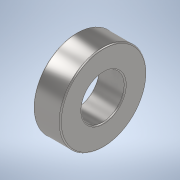
# Autodesk Inventor part: 608zz-bearing
Saved by Autodesk Inventor 2020 (Build 240168000, 168)
## iProperties
Created: 2021-03-01
Part Number: 608zz-bearing
Material: Steel, Carbon
Document SubType Name: Modeling
Designer: AOB
Mass: 5.9086 g
Surface Area: 6.6564 cm^2
Volume: 0.752688 cm^3
Density: 7.85 g/cm^3
Appearance: Semi-Polished
Author: AOB
Autodesk Inventor part; units mm, degrees
ref_plane "YZ Plane" through (0, 0, 0) normal (1, 0, 0) x (0, 1, 0)
ref_plane "XZ Plane" through (0, 0, 0) normal (0, 1, 0) x (-1, 0, 0)
ref_plane "XY Plane" through (0, 0, 0) normal (0, 0, 1) x (1, 0, 0)
sketch "Sketch1" plane through (0, 0, 0) normal (0, 0, 1) x (1, 0, 0)
  line L0 (0.2, 0) -> (4.8, 0)
  line L1 (5, -0.2) -> (5, -3.8)
  line L2 (4.8, -4) -> (0.2, -4)
  line L3 (0, -3.8) -> (0, -0.2)
  arc A0 (0.2, 0) -> (0, -0.2) centre (0.2, -0.2) ccw
  arc A1 (5, -0.2) -> (4.8, 0) centre (4.8, -0.2) ccw
  arc A2 (4.8, -4) -> (5, -3.8) centre (4.8, -3.8) ccw
  arc A3 (0, -3.8) -> (0.2, -4) centre (0.2, -3.8) ccw
  line L4 (0, -8) -> (5.8004, -8)
  point P0 (0, 0)
  point P1 (5, -4)
  point P2 (5, 0)
  dimension "d0" = 5
  dimension "d1" = 4
  dimension "d2" = 0.2
  dimension "d3" = 4
  constraints: 10 end point, 8 point on circle, 8 tangent, 6 point on line, 4 centre point, 3 equal radius, 2 horizontal, 2 parallel, 1 perpendicular
  measures "d0" distance of point (0, 0) point (5, 0)
  measures "d1" distance of point (5, 0) point (5, -4)
  measures "d2" radius of A0
  measures "d3" distance from line of L2 L4.end
revolve "Revolution1" add sketch "Sketch1" angle 360 about axis through (0, -8, 0) along (1, 0, 0)
body "Solid1"
